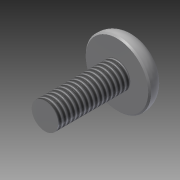
# Autodesk Inventor part: 10-32 Bolt
Saved by Autodesk Inventor 2013 (Build 170138000, 138)
## iProperties
Created: 2013-03-11
Part Number: 10-32 Bolt
Material: Steel
Document SubType Name: Modeling
Designer: Moses
Mass: 3.6373 g
Surface Area: 4.93821 cm^2
Volume: 0.46335 cm^3
Density: 7.85 g/cm^3
Author: Moses
Autodesk Inventor part; units mm, degrees
ref_plane "YZ Plane" through (0, 0, 0) normal (1, 0, 0) x (0, 1, 0)
ref_plane "XZ Plane" through (0, 0, 0) normal (0, 1, 0) x (-1, 0, 0)
ref_plane "XY Plane" through (0, 0, 0) normal (0, 0, 1) x (1, 0, 0)
sketch "Sketch1" plane through (0, 0, 0) normal (0, 0, 1) x (1, 0, 0)
  circle A0 centre (0, 0) radius 5.763
  circle A1 centre (0, 0) radius 2.3495
  line L0 (2.8868, 0) -> (1.4434, -2.5)
  line L1 (1.4434, -2.5) -> (-1.4434, -2.5)
  line L2 (-1.4434, -2.5) -> (-2.8868, 0)
  line L3 (-2.8868, 0) -> (-1.4434, 2.5)
  line L4 (-1.4434, 2.5) -> (1.4434, 2.5)
  line L5 (1.4434, 2.5) -> (2.8868, 0)
  dimension "d0" = 11.526
  dimension "d2" = 4.699
  dimension "d5" = 5
  constraints: 12 end point, 3 coincident, 2 centre point, 1 horizontal, 13 other
  measures "d0" diameter of A0
  measures "d2" diameter of A1
  measures "d5" distance between parallel lines of L1 L4
extrude "Extrusion1" add sketch "Sketch1" along normal blind 12.7 contours A1
extrude "Extrusion2" add sketch "Sketch1" against normal blind 3.175 contours A0 | A1 | L0 L1 L2 L3 L4 L5
fillet "Fillet1" radius 2.54 1 edges at (-5.763, 0, -3.175)
sketch "Sketch2" plane through (0, 0, -3.175) normal (0, 0, -1) x (-1, 0, 0)
  circle A0 centre (0, 0) radius 2.3495 projected
  circle A1 centre (0, 0) radius 3.223 projected
  line L0 (2.8868, 0) -> (1.4434, -2.5)
  line L1 (1.4434, -2.5) -> (-1.4434, -2.5)
  line L2 (-1.4434, -2.5) -> (-2.8868, 0)
  line L3 (-2.8868, 0) -> (-1.4434, 2.5)
  line L4 (-1.4434, 2.5) -> (1.4434, 2.5)
  line L5 (1.4434, 2.5) -> (2.8868, 0)
  dimension "d9" = 5
  constraints: 12 end point, 1 coincident, 1 horizontal, 13 other
  measures "d9" distance between parallel lines of L1 L4
extrude "Extrusion3" cut sketch "Sketch2" against normal blind 1.905 contours A0 | L0 L1 L2 L3 L4 L5
thread "Thread1" size "10-32 UNF" class "2A" standard "ANSI Unified Screw Threads" full length
chamfer "Chamfer1" distance 0.254 angle 45 7 edges at (2.1651, 1.25, -3.175) (0, 2.5, -3.175) (-2.1651, 1.25, -3.175) (2.1651, -1.25, -3.175) (0, -2.5, -3.175) (-2.1651, -1.25, -3.175) (-5.763, 0, 0)
body "Solid1"
